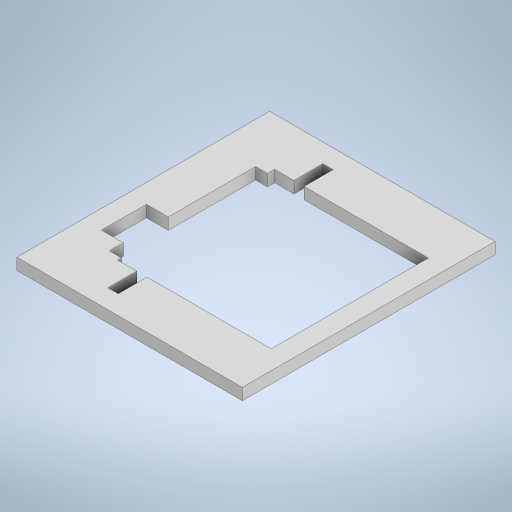
# Autodesk Inventor part: ft5330m_profile_v2
Saved by Autodesk Inventor 2023.1 (Build 271208000, 208)
## iProperties
Created: 2026-05-19
Part Number: ft5330m_profile_v2
Material: Generic
Document SubType Name: Modeling
Designer: Lars
Density: 1 g/cm^3
Appearance: Default
Author: Lars
Autodesk Inventor part; units mm, degrees
ref_plane "YZ Plane" through (0, 0, 0) normal (1, 0, 0) x (0, 1, 0)
ref_plane "XZ Plane" through (0, 0, 0) normal (0, 1, 0) x (-1, 0, 0)
ref_plane "XY Plane" through (0, 0, 0) normal (0, 0, 1) x (1, 0, 0)
sketch "Sketch1" plane through (0, 0, 0) normal (0, 1, 0) x (-1, 0, 0)
  line L0 (0, 0) -> (32.08, 0)
  line L1 (39.5, 0) -> (39.5, -1)
  line L2 (39.5, -40.4) -> (34.5, -40.4)
  line L3 (0, -40.4) -> (0, 0)
  line L4 (39.5, -20.2) -> (34.5, -20.2) construction
  line L5 (34.5, 7.45) -> (32.08, 7.45)
  line L6 (32.08, 7.45) -> (32.08, 0)
  line L7 (32.08, -47.85) -> (34.5, -47.85)
  line L8 (34.5, -47.85) -> (34.5, -40.4)
  line L9 (42.6, -1) -> (39.5, -1)
  line L10 (39.5, -1) -> (39.5, -38.55) construction
  line L11 (39.5, -38.55) -> (42.6, -38.55)
  line L12 (42.6, -38.55) -> (42.6, -16.01)
  line L13 (48.25, -4.61) -> (42.6, -4.61)
  line L14 (42.6, -4.61) -> (42.6, -16.01) construction
  line L15 (42.6, -16.01) -> (48.25, -16.01)
  line L16 (48.25, -16.01) -> (48.25, -4.61)
  line L17 (48.25, 7.45) -> (0, 7.45) construction
  line L18 (0, 7.45) -> (0, -47.85) construction
  line L19 (0, -47.85) -> (48.25, -47.85) construction
  line L20 (48.25, -47.85) -> (48.25, 7.45) construction
  line L21 (-5, 12.45) -> (53.25, 12.45)
  line L22 (53.25, 12.45) -> (53.25, -52.85)
  line L23 (53.25, -52.85) -> (-5, -52.85)
  line L24 (-5, -52.85) -> (-5, 12.45)
  line L25 (34.5, 0) -> (39.5, 0)
  line L26 (32.08, 0) -> (34.5, 0) construction
  line L27 (34.5, -40.4) -> (32.08, -40.4) construction
  line L28 (32.08, -40.4) -> (0, -40.4)
  line L29 (39.5, -1) -> (39.5, -38.55) construction
  line L30 (39.5, -38.55) -> (39.5, -40.4)
  line L31 (42.6, -4.61) -> (42.6, -1)
  line L32 (42.6, -16.01) -> (42.6, -4.61) construction
  line L33 (32.08, 0) -> (32.08, -40.4) construction
  line L34 (34.5, 0) -> (34.5, 7.45)
  line L35 (34.5, -40.4) -> (34.5, 0) construction
  line L36 (32.08, -40.4) -> (32.08, -47.85)
  line L37 (34.6, 7.55) -> (31.98, 7.55)
  line L38 (31.98, 7.55) -> (31.98, 0.1)
  line L39 (31.98, 0.1) -> (-0.1, 0.1)
  line L40 (-0.1, 0.1) -> (-0.1, -40.5)
  line L41 (-0.1, -40.5) -> (31.98, -40.5)
  line L42 (31.98, -40.5) -> (31.98, -47.95)
  line L43 (31.98, -47.95) -> (34.6, -47.95)
  line L44 (34.6, -47.95) -> (34.6, -40.5)
  line L45 (34.6, -40.5) -> (39.6, -40.5)
  line L46 (39.6, -40.5) -> (39.6, -38.65)
  line L47 (39.6, -38.65) -> (42.7, -38.65)
  line L48 (42.7, -38.65) -> (42.7, -16.11)
  line L49 (42.7, -16.11) -> (48.35, -16.11)
  line L50 (48.35, -16.11) -> (48.35, -4.51)
  line L51 (48.35, -4.51) -> (42.7, -4.51)
  line L52 (42.7, -4.51) -> (42.7, -0.9)
  line L53 (42.7, -0.9) -> (39.6, -0.9)
  line L54 (39.6, -0.9) -> (39.6, 0.1)
  line L55 (39.6, 0.1) -> (34.6, 0.1)
  line L56 (34.6, 0.1) -> (34.6, 7.55)
  point P0 (41.05, -1)
  point P1 (42.6, -10.31)
  point P2 (33.29, -47.85)
  point P3 (48.25, -10.31)
  point P4 (33.29, 7.45)
  point P5 (0, -20.2)
  dimension "d0" = 39.5
  dimension "d1" = 40.4
  dimension "d2" = 5
  dimension "d3" = 2.42
  dimension "d4" = 55.3
  dimension "d5" = 3.1
  dimension "d6" = 37.55
  dimension "d8" = 5.65
  dimension "d9" = 11.4
  dimension "d10" = 4.61
  dimension "d11" = 5
  dimension "d12" = 0.1
  constraints: 114 end point, 45 parallel, 22 perpendicular, 8 horizontal, 8 midpoint, 6 point on line, 22 other
  measures "d0" distance of L2.start L3.start
  measures "d1" distance of L1.start L2.start
  measures "d2" distance of L4.end L4.start
  measures "d3" distance of L7.end L7.start
  measures "d4" distance of L7.start L5.end
  measures "d5" distance of L11.end L10.end
  measures "d6" distance of L10.end L1.end
  measures "d8" distance of L15.end L12.end
  measures "d9" distance of L12.end L13.end
  measures "d10" distance between parallel lines of L13 L0
  measures "d11" distance between parallel lines of L17 L21
  measures "d12" distance between parallel lines of L34 L56
extrude "Extrusion1" add sketch "Sketch1" along normal blind 3 contours L21 L22 L23 L24
body "Solid1"
